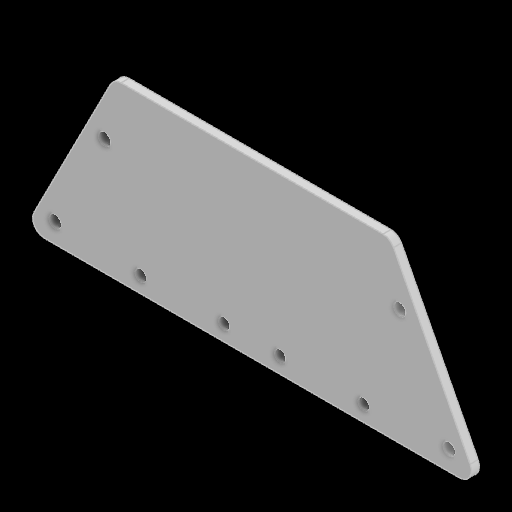
# Autodesk Inventor part: BreakerMount
Saved by Autodesk Inventor 2025.2 (Build 292293000, 293)
## iProperties
Created: 2025-11-18
Part Number: BreakerMount
Material: Generic
Document SubType Name: Sheet Metal
Designer: valer
Density: 1 g/cm^3
Sheet Metal Rule: Default
Appearance: Default
Author: valer
Autodesk Inventor part; units mm, degrees
ref_plane "YZ Plane" through (0, 0, 0) normal (1, 0, 0) x (0, 1, 0)
ref_plane "XZ Plane" through (0, 0, 0) normal (0, 1, 0) x (-1, 0, 0)
ref_plane "XY Plane" through (0, 0, 0) normal (0, 0, 1) x (1, 0, 0)
sketch "Base" plane through (0, 0, 0) normal (0, 0, 1) x (1, 0, 0)
  line L0 (0, 0) -> (70.3402, 0)
  line L1 (70.3402, 0) -> (115.4849, -88)
  line L2 (115.4849, -88) -> (0, -88)
  line L3 (0, -88) -> (0, 0) construction
  line L4 (0, 0) -> (-70.3402, 0)
  line L5 (-70.3402, 0) -> (-115.4849, -88)
  line L6 (-115.4849, -88) -> (0, -88)
  line L7 (-63.3831, 22.3248) -> (-182.4251, -209.7225) construction
  dimension "d1" = 88
  dimension "d3" = 4
  measures "d1" distance between parallel lines of L6 L4
  measures "d3" distance between parallel lines of L7 L5
extrude "Plate1" add sketch "Base" along normal blind 4
fillet "FilletsFeature" radius 6 4 edges at (-70.3402, 0, 2) (70.3402, 0, 2) (115.4849, -88, 2) (-115.4849, -88, 2)
sketch "BreakerMounts" plane through (0, 0, 0) normal (0, 0, -1) x (-1, 0, 0)
  circle A0 centre (56.75, -80) radius 2.75 projected
  circle A1 centre (14.25, -80) radius 2.75 projected
  circle A2 centre (-14.25, -80) radius 2.75 projected
  circle A3 centre (-56.75, -80) radius 2.75 projected
  point P0 (0, 0)
extrude "BreakerMountsFeature" cut sketch "BreakerMounts" against normal blind 4
sketch "FrameMounts" plane through (0, 0, 0) normal (0, 0, -1) x (-1, 0, 0)
  circle A0 centre (100.2396, -78) radius 3
  circle A1 centre (75.1349, -29.0638) radius 3
  line L0 (100.2396, -78) -> (75.1349, -29.0638) construction
  line L1 (72.0133, -3.2613) -> (111.0019, -79.2613) construction
  line L2 (105.6634, -88) -> (-105.6634, -88) projected
  line L3 (0, -105.6) -> (0, 17.6) construction
  circle A2 centre (-100.2396, -78) radius 3
  circle A3 centre (-75.1349, -29.0638) radius 3
  point P0 (0, 0)
  dimension "d6" = 6
  dimension "d7" = 6
  dimension "d8" = 10
  dimension "d9" = 9
  dimension "d10" = 55
  constraints: 4 centre point, 2 end point, 2 symmetric about line, 1 parallel, 2 other
  measures "d6" diameter of A0
  measures "d7" diameter of A1
  measures "d8" distance from line of L2 L0.start
  measures "d9" distance between parallel lines of L1 L0
  measures "d10" distance of L0.start L0.end
extrude "FrameMountsFeature" cut sketch "FrameMounts" against normal blind 4
equation "\"d4\" = Thickness"
equation "\"d11\" = Thickness"
equation "\"d0\" = Thickness"
equation "\"BendRadius\" = Thickness"
equation "\"BendReliefWidth\" = Thickness"
equation "\"BendReliefDepth\" = 0.5 * Thickness"
equation "\"CornerReliefSize\" = 4 * Thickness"
equation "\"MinimumRemnant\" = 2 * Thickness"
equation "\"TransitionRadius\" = BendRadius"
equation "\"JacobiRadiusSize\" = BendRadius"
equation "\"GapSize\" = Thickness"
equation "\"Thickness\" = 4"
body "Solid1"
